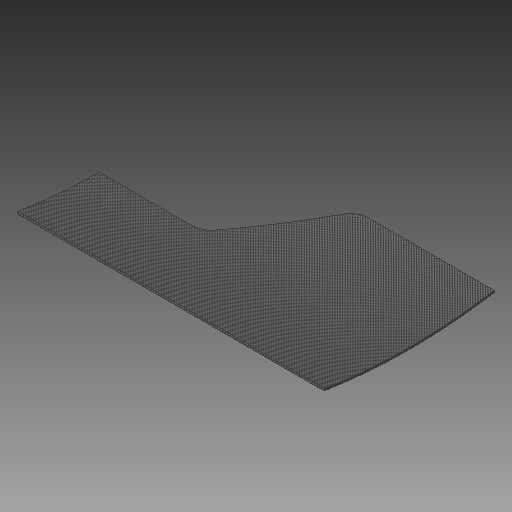
# Autodesk Inventor part: type7_element_base
Saved by Autodesk Inventor 2018.1 (Build 221171000, 171)
## iProperties
Created: 2017-11-03
Part Number: type7_element_base
Material: CFRP
Document SubType Name: Modeling
Designer: ku_sk
Density: 1.43 g/cm^3
Appearance: カーボンファイバー
Mass: 371.961 g
Surface Area: 1774.02 cm^2
Volume: 260.112 cm^3
Author: ku_sk
Autodesk Inventor part; units mm, degrees
ref_plane "YZ Plane" through (0, 0, 0) normal (1, 0, 0) x (0, 1, 0)
ref_plane "XZ Plane" through (0, 0, 0) normal (0, 1, 0) x (-1, 0, 0)
ref_plane "XY Plane" through (0, 0, 0) normal (0, 0, 1) x (1, 0, 0)
sketch "スケッチ1" plane through (0, 0, 0) normal (1, 0, 0) x (0, 1, 0)
  arc A0 (7.0384, 125) -> (7.0384, -125) centre (780.277, 0) ccw
  arc A1 (10, 124.5212) -> (10, -124.5212) centre (780.277, 0) ccw
  line L0 (10, 124.5212) -> (7.0384, 125)
  line L1 (10, -124.5212) -> (7.0384, -125)
  line L2 (0, -175) -> (0, 175) projected
  line L3 (10, 124.5212) -> (10, -124.5212)
  point P0 (0, 0)
  point P1 (0, 0)
  dimension "d0" = 3
  dimension "d1" = 250
  dimension "d2" = 10
  constraints: 6 end point, 5 point on circle, 4 line through centre, 2 centre point, 1 coincident, 1 concentric, 1 parallel, 1 tangent
  measures "d0" distance of L0.start L0.end
  measures "d1" distance of L1.end L0.end
  measures "d2" distance between parallel lines of L2 L3
extrude "押し出し1" add sketch "スケッチ1" along normal mid plane 450 contours L0 A1 L2 A0 | L2 A0 | L2 A1 L1 A0
sketch "スケッチ2" plane through (0, 0, 0) normal (0, 1, 0) x (-1, 0, 0)
  line L0 (75, 5) -> (225, 5)
  line L1 (225, -125) -> (-225, -125) projected
  line L2 (225, 124.5212) -> (225, -124.5212) projected
  line L3 (225, -124.5212) -> (-225, -124.5212) projected
  line L4 (-225, 125) -> (225, 125) projected
  line L5 (75, 5) -> (-25, -125)
  line L6 (-225, -124.5212) -> (-225, 124.5212) projected
  line L7 (225, 5) -> (225, -125)
  line L8 (-25, -125) -> (225, -125)
  point P0 (0, 0)
  dimension "d5" = 120
  dimension "d6" = 200
  dimension "d7" = 300
  constraints: 8 end point, 2 point on line, 1 collinear, 1 parallel, 1 perpendicular
  measures "d5" distance between parallel lines of L4 L0
  measures "d6" distance from line of L6 L5.end
  measures "d7" distance from line of L6 L0.start
extrude "押し出し2" cut sketch "スケッチ2" along normal through all both and the other way through all
fillet "フィレット1" radius 30 2 edges at (-75, -1.484, 5) (24.8159, 8.5192, -124.7606)
